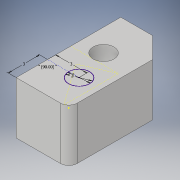
# Autodesk Inventor part: testpart
Saved by Autodesk Inventor 2018 (Build 220112000, 112)
## iProperties
Created: 2017-09-14
Part Number: testpart
Material: Generic
Document SubType Name: Modeling
Designer: SWCbootcamp
Density: 1 g/cm^3
Appearance: Default
Author: SWCbootcamp
Autodesk Inventor part; units mm, degrees
ref_plane "YZ Plane" through (0, 0, 0) normal (1, 0, 0) x (0, 1, 0)
ref_plane "XZ Plane" through (0, 0, 0) normal (0, 1, 0) x (-1, 0, 0)
ref_plane "XY Plane" through (0, 0, 0) normal (0, 0, 1) x (1, 0, 0)
sketch "Sketch1" plane through (0, 0, 0) normal (0, 1, 0) x (-1, 0, 0)
  line L0 (0, 0) -> (5.031, 0)
  line L1 (5.031, 0) -> (5.031, -10)
  line L2 (5.031, -10) -> (0, -10)
  line L3 (0, -10) -> (0, 0)
  dimension "d0" = 10
  constraints: 8 end point, 2 parallel, 1 horizontal, 1 perpendicular
  measures "d0" distance of L0.end L1.end
extrude "Extrusion1" add sketch "Sketch1" along normal blind 5
sketch "Sketch2" plane through (0, 5, 0) normal (0, 1, 0) x (1, 0, 0)
  point P0 (0, 0)
sketch "Sketch3" plane through (0, 5, 0) normal (0, 1, 0) x (1, 0, 0)
  circle A0 centre (-2.8935, 6.2146) radius 1
  point P0 (0, 0)
  dimension "d14" = 2
  constraints: 1 centre point
  measures "d14" diameter of A0
extrude "Extrusion2" cut sketch "Sketch3" against normal blind 5
fillet "Fillet1" radius 0.8 1 edges at (0, 2.5, 0)
chamfer "Chamfer1" distance 2 angle 45 1 edges at (0, 2.5, -10)
sketch "Sketch4" plane through (0, 5, 0) normal (0, 1, 0) x (1, 0, 0)
  line L0 (-5.031, 0) -> (-0.8, 0) construction
  line L1 (-5.031, 0) -> (-5.031, 5.2141) construction
  line L2 (-5.031, 5.2141) -> (-0.484, 5.2141) construction
  line L3 (-0.484, 5.2141) -> (-0.484, 0) construction
  line L4 (-0.484, 0) -> (-3.3034, 3.9743) construction
  line L5 (-3.3034, 3.9743) -> (-0.484, 5.2141) construction
  line L6 (-5.031, 0) -> (-5.031, 3) construction
  line L7 (-5.031, 10) -> (-5.031, 0) construction
  line L8 (-5.031, 3) -> (-2.031, 3) construction
  circle A0 centre (-2.031, 3) radius 1 construction
  circle A1 centre (-2.031, 3) radius 1
  point P0 (0, 0)
  dimension "d9" = 3
  dimension "d10" = 3
  dimension "d11" = 90
  dimension "d12" = 2
  dimension "d13" = 2
  constraints: 14 end point, 3 perpendicular, 2 centre point, 2 coincident, 1 point on line, 1 vertical
  measures "d9" distance of L0.start L6.end
  measures "d10" distance of L6.end L8.end
  measures "d11" angle of L6 L8
  measures "d12" diameter of A0
  measures "d13" diameter of A1
body "Solid1"
